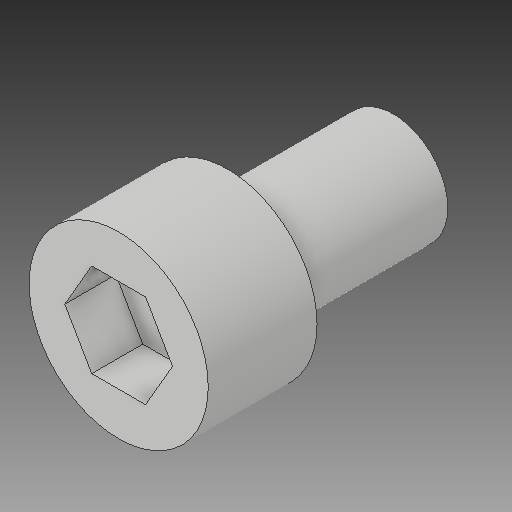
# Autodesk Inventor part: shcs-8-0250
Saved by Autodesk Inventor 2017 (Build 210142000, 142)
## iProperties
Created: 2016-07-01
Part Number: shcs-8-0250
Material: Generic
Document SubType Name: Modeling
Designer: rickab1
Density: 1 g/cm^3
Appearance: Default
Author: rickab1
Autodesk Inventor part; units mm, degrees
ref_plane "YZ Plane" through (0, 0, 0) normal (1, 0, 0) x (0, 1, 0)
ref_plane "XZ Plane" through (0, 0, 0) normal (0, 1, 0) x (-1, 0, 0)
ref_plane "XY Plane" through (0, 0, 0) normal (0, 0, 1) x (1, 0, 0)
sketch "Sketch1" plane through (0, 0, 0) normal (0, 0, 1) x (1, 0, 0)
  circle A0 centre (0, 0) radius 3.429
  dimension "head_dia" = 6.858
  constraints: 1 centre point, 1 coincident
  measures "head_dia" diameter of A0
extrude "Extrusion1" add sketch "Sketch1" against normal blind 4.1656
sketch "Sketch2" plane through (0, 0, -4.1656) normal (0, 0, -1) x (-1, 0, 0)
  circle A0 centre (0, 0) radius 2.0828
  dimension "body_dia" = 4.1656
  constraints: 1 centre point, 1 coincident
  measures "body_dia" diameter of A0
extrude "Extrusion2" add sketch "Sketch2" along normal blind 6.35
sketch "Sketch3" plane through (0, 0, 0) normal (0, 0, 1) x (1, 0, 0)
  line L0 (2.0622, 0) -> (1.0311, -1.7859)
  line L1 (1.0311, -1.7859) -> (-1.0311, -1.7859)
  line L2 (-1.0311, -1.7859) -> (-2.0622, 0)
  line L3 (-2.0622, 0) -> (-1.0311, 1.7859)
  line L4 (-1.0311, 1.7859) -> (1.0311, 1.7859)
  line L5 (1.0311, 1.7859) -> (2.0622, 0)
  point P0 (0, 0)
  point P1 (0, 0)
  dimension "allen" = 3.5719
  constraints: 12 end point, 1 coincident, 1 horizontal alignment, 13 other
  measures "allen" distance between parallel lines of L1 L4
extrude "Extrusion3" cut sketch "Sketch3" against normal blind 1.9558
body "Solid1"
